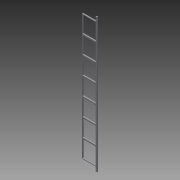
# Autodesk Inventor part: Gesims
Saved by Autodesk Inventor 2015 (Build 190159000, 159)
## iProperties
Created: 2015-09-16
Part Number: Gesims
Material: Generic
Document SubType Name: Modeling
Designer: Simen
Density: 1 g/cm^3
Appearance: Default
Author: Simen
Autodesk Inventor part; units mm, degrees
ref_plane "YZ Plane" through (0, 0, 0) normal (1, 0, 0) x (0, 1, 0)
ref_plane "XZ Plane" through (0, 0, 0) normal (0, 1, 0) x (-1, 0, 0)
ref_plane "XY Plane" through (0, 0, 0) normal (0, 0, 1) x (1, 0, 0)
sketch "Sketch1" plane through (0, 0, 0) normal (0, 1, 0) x (-1, 0, 0)
  line L0 (0, 0) -> (100, 0)
  line L1 (100, 0) -> (100, -360)
  line L2 (100, -360) -> (1260, -360)
  line L3 (1260, -360) -> (1260, -10860)
  line L4 (1260, -10860) -> (100, -10860)
  line L5 (100, -10860) -> (100, -11220)
  line L6 (100, -11220) -> (0, -11220)
  line L7 (0, -11220) -> (0, 0)
  dimension "d0" = 11220
  dimension "d1" = 100
  dimension "d2" = 100
  dimension "d3" = 1260
  dimension "d4" = 10500
  dimension "d5" = 360
  constraints: 16 end point, 7 perpendicular, 1 horizontal
  measures "d0" distance between parallel lines of L6 L0
  measures "d1" distance between parallel lines of L7 L1
  measures "d2" distance between parallel lines of L7 L5
  measures "d3" distance between parallel lines of L3 L7
  measures "d4" distance between parallel lines of L4 L2
  measures "d5" distance between parallel lines of L0 L2
extrude "Extrusion1" add sketch "Sketch1" along normal blind 100
sketch "Sketch2" plane through (0, 100, 0) normal (0, 1, 0) x (1, 0, 0)
  line L0 (-1210, 410) -> (-100, 410)
  line L1 (-100, 410) -> (-100, 1810)
  line L2 (-100, 1810) -> (-1210, 1810)
  line L3 (-1210, 1810) -> (-1210, 410)
  point P0 (0, 0)
  dimension "d14" = 1400
  dimension "d15" = 1110
  dimension "d16" = 100
  dimension "d17" = 410
  constraints: 8 end point, 2 parallel, 1 horizontal, 1 perpendicular
  measures "d14" distance between parallel lines of L2 L0
  measures "d15" distance between parallel lines of L3 L1
  measures "d16" distance from line of point (0, 0) L1
  measures "d17" distance from line of point (0, 0) L0
extrude "Extrusion2" cut sketch "Sketch2" against normal blind 100
sketch "Sketch3" plane through (0, 100, 0) normal (0, 1, 0) x (1, 0, 0)
  line L0 (-1210, 1910) -> (-100, 1910)
  line L1 (-100, 1910) -> (-100, 3310)
  line L2 (-100, 3310) -> (-1210, 3310)
  line L3 (-1210, 3310) -> (-1210, 1910)
  point P0 (0, 0)
  dimension "d20" = 1910
  dimension "d21" = 100
  dimension "d22" = 1400
  dimension "d23" = 1110
  constraints: 8 end point, 2 parallel, 1 horizontal, 1 perpendicular
  measures "d20" vertical distance of L0.end point (0, 0)
  measures "d21" horizontal distance of point (0, 0) L0.end
  measures "d22" distance between parallel lines of L2 L0
  measures "d23" distance between parallel lines of L1 L3
extrude "Extrusion3" cut sketch "Sketch3" against normal blind 100
sketch "Sketch4" plane through (0, 100, 0) normal (0, 1, 0) x (1, 0, 0)
  line L0 (-1210, 3410) -> (-100, 3410)
  line L1 (-100, 3410) -> (-100, 4810)
  line L2 (-100, 4810) -> (-1210, 4810)
  line L3 (-1210, 4810) -> (-1210, 3410)
  point P0 (0, 0)
  dimension "d26" = 3410
  dimension "d27" = 100
  dimension "d28" = 1400
  dimension "d29" = 1110
  constraints: 8 end point, 2 parallel, 1 horizontal, 1 perpendicular
  measures "d26" vertical distance of L0.end point (0, 0)
  measures "d27" horizontal distance of L0.end point (0, 0)
  measures "d28" distance between parallel lines of L2 L0
  measures "d29" distance between parallel lines of L1 L3
extrude "Extrusion5" cut sketch "Sketch4" against normal blind 100
sketch "Sketch5" plane through (0, 100, 0) normal (0, 1, 0) x (1, 0, 0)
  line L0 (-1210, 4910) -> (-100, 4910)
  line L1 (-100, 4910) -> (-100, 6310)
  line L2 (-100, 6310) -> (-1210, 6310)
  line L3 (-1210, 6310) -> (-1210, 4910)
  point P0 (0, 0)
  dimension "d37" = 4910
  dimension "d38" = 100
  dimension "d39" = 1400
  dimension "d40" = 1110
  constraints: 8 end point, 2 parallel, 1 horizontal, 1 perpendicular
  measures "d37" vertical distance of point (0, 0) L0.end
  measures "d38" horizontal distance of point (0, 0) L0.end
  measures "d39" distance between parallel lines of L2 L0
  measures "d40" distance between parallel lines of L1 L3
extrude "Extrusion6" cut sketch "Sketch5" against normal blind 100
sketch "Sketch6" plane through (0, 100, 0) normal (0, 1, 0) x (1, 0, 0)
  line L0 (-1210, 6410) -> (-100, 6410)
  line L1 (-100, 6410) -> (-100, 7810)
  line L2 (-100, 7810) -> (-1210, 7810)
  line L3 (-1210, 7810) -> (-1210, 6410)
  point P0 (0, 0)
  dimension "d43" = 1400
  dimension "d44" = 1110
  dimension "d45" = 6410
  dimension "d46" = 100
  constraints: 8 end point, 2 parallel, 1 horizontal, 1 perpendicular
  measures "d43" distance between parallel lines of L2 L0
  measures "d44" distance between parallel lines of L1 L3
  measures "d45" vertical distance of L0.end point (0, 0)
  measures "d46" horizontal distance of point (0, 0) L0.end
extrude "Extrusion7" cut sketch "Sketch6" against normal blind 100
sketch "Sketch7" plane through (0, 100, 0) normal (0, 1, 0) x (1, 0, 0)
  line L0 (-1210, 7910) -> (-100, 7910)
  line L1 (-100, 7910) -> (-100, 9310)
  line L2 (-100, 9310) -> (-1210, 9310)
  line L3 (-1210, 9310) -> (-1210, 7910)
  point P0 (0, 0)
  dimension "d49" = 1400
  dimension "d50" = 1110
  dimension "d51" = 7910
  dimension "d52" = 100
  constraints: 8 end point, 2 parallel, 1 horizontal, 1 perpendicular
  measures "d49" distance of L1.end L0.end
  measures "d50" distance between parallel lines of L1 L3
  measures "d51" vertical distance of point (0, 0) L0.end
  measures "d52" horizontal distance of point (0, 0) L0.end
extrude "Extrusion8" cut sketch "Sketch7" against normal blind 100
sketch "Sketch8" plane through (0, 100, 0) normal (0, 1, 0) x (1, 0, 0)
  line L0 (-1210, 9410) -> (-100, 9410)
  line L1 (-100, 9410) -> (-100, 10810)
  line L2 (-100, 10810) -> (-1210, 10810)
  line L3 (-1210, 10810) -> (-1210, 9410)
  point P0 (0, 0)
  dimension "d55" = 1110
  dimension "d56" = 1400
  dimension "d57" = 9410
  dimension "d58" = 100
  constraints: 8 end point, 2 parallel, 1 horizontal, 1 perpendicular
  measures "d55" distance of L2.end L1.end
  measures "d56" distance of L1.end L0.end
  measures "d57" vertical distance of point (0, 0) L0.end
  measures "d58" horizontal distance of point (0, 0) L0.end
extrude "Extrusion9" cut sketch "Sketch8" against normal blind 100
body "Solid1"
